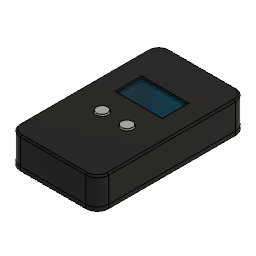
sms-telegram-enclosure (Autodesk Fusion 360 design; units mm, degrees)
part number: 2026-09-10-15-50-54-312
Autodesk Fusion 360 part; units mm, degrees
sketch "cover_outline" plane through (0, 0, 0) normal (0, 0, 1) x (1, 0, 0)
  line L0 (23, 78) -> (-23, 78)
  line L1 (-23, 78) -> (-23, 0)
  line L2 (-23, 0) -> (23, 0)
  line L3 (23, 0) -> (23, 78)
extrude "Extrude1" add sketch "cover_outline" along normal blind 2 makes body 1
fillet "Fillet1" radius 6 4 edges at (23, 0, 1) (-23, 0, 1) (-23, 78, 1) (23, 78, 1) on bodies 1
ref_plane "WorkPlane1" through (0, 0, 2) normal (0, 0, 1) x (1, 0, 0)
sketch "cover_m6" plane through (0, 0, 2) normal (0, 0, 1) x (1, 0, 0)
  circle A0 centre (-17, 72) radius 3.2
  circle A1 centre (17, 72) radius 3.2
  circle A2 centre (-17, 32) radius 3.2
  circle A3 centre (17, 32) radius 3.2
ref_plane "WorkPlane2" through (0, 0, 2) normal (0, 0, 1) x (1, 0, 0)
sketch "shell_outline" plane through (0, 0, 2) normal (0, 0, 1) x (1, 0, 0)
  line L0 (23, 78) -> (-23, 78)
  line L1 (-23, 78) -> (-23, 0)
  line L2 (-23, 0) -> (23, 0)
  line L3 (23, 0) -> (23, 78)
extrude "Extrude3" add sketch "shell_outline" along normal blind 14 separate body makes body 2
fillet "Fillet2" radius 6 4 edges at (23, 0, 9) (-23, 0, 9) (-23, 78, 9) (23, 78, 9) on bodies 2
shell "Shell1" thickness 2 removed faces 1 at (-7.6667, 50, 2) on bodies 2
ref_plane "WorkPlane3" through (0, 0, 2) normal (0, 0, 1) x (1, 0, 0)
sketch "pillars" plane through (0, 0, 2) normal (0, 0, 1) x (1, 0, 0)
  circle A0 centre (-17, 72) radius 6
  circle A1 centre (17, 72) radius 6
  circle A2 centre (-17, 32) radius 6
  circle A3 centre (17, 32) radius 6
ref_plane "WorkPlane4" through (0, 0, 2) normal (0, 0, 1) x (1, 0, 0)
sketch "insert_holes" plane through (0, 0, 2) normal (0, 0, 1) x (1, 0, 0)
  circle A0 centre (-17, 72) radius 4
  circle A1 centre (17, 72) radius 4
  circle A2 centre (-17, 32) radius 4
  circle A3 centre (17, 32) radius 4
ref_plane "WorkPlane5" through (0, 78, 0) normal (0, 1, 0) x (0, 0, 1)
sketch "usb_c" plane through (0, 78, 0) normal (0, 1, 0) x (1, 0, 0)
  line L0 (4.6, -7.9) -> (-4.6, -7.9)
  line L1 (-4.6, -7.9) -> (-4.6, -4.3)
  line L2 (-4.6, -4.3) -> (4.6, -4.3)
  line L3 (4.6, -4.3) -> (4.6, -7.9)
extrude "Extrude6" cut sketch "usb_c" along normal mid plane 3 bodies 2
ref_plane "WorkPlane6" through (0, 0, 16) normal (0, 0, 1) x (1, 0, 0)
sketch "front_ui" plane through (0, 0, 16) normal (0, 0, 1) x (1, 0, 0)
  line L0 (12.25, 58.4) -> (-12.25, 58.4)
  line L1 (-12.25, 58.4) -> (-12.25, 44.6)
  line L2 (-12.25, 44.6) -> (12.25, 44.6)
  line L3 (12.25, 44.6) -> (12.25, 58.4)
  circle A0 centre (-6.5, 32) radius 3.1
  circle A1 centre (6.5, 32) radius 3.1
extrude "Extrude7" cut sketch "front_ui" against normal blind 2.6 bodies 2
ref_plane "WorkPlane7" through (0, 0, 3.5) normal (0, 0, 1) x (1, 0, 0)
sketch "XIAO_pcb_sk" plane through (0, 0, 3.5) normal (0, 0, 1) x (1, 0, 0)
  line L0 (-10.5, 58) -> (10.5, 58)
  line L1 (10.5, 58) -> (10.5, 75.5)
  line L2 (10.5, 75.5) -> (-10.5, 75.5)
  line L3 (-10.5, 75.5) -> (-10.5, 58)
extrude "Extrude8" add sketch "XIAO_pcb_sk" along normal blind 1 separate body makes body 3
ref_plane "WorkPlane8" through (0, 0, 2.5) normal (0, 0, 1) x (1, 0, 0)
sketch "XIAO_bottom_sk" plane through (0, 0, 2.5) normal (0, 0, 1) x (1, 0, 0)
  line L0 (-9, 60) -> (9, 60)
  line L1 (9, 60) -> (9, 74)
  line L2 (9, 74) -> (-9, 74)
  line L3 (-9, 74) -> (-9, 60)
extrude "Extrude9" add sketch "XIAO_bottom_sk" along normal blind 1 separate body makes body 4
ref_plane "WorkPlane9" through (0, 0, 4.5) normal (0, 0, 1) x (1, 0, 0)
sketch "XIAO_shield_sk" plane through (0, 0, 4.5) normal (0, 0, 1) x (1, 0, 0)
  line L0 (-6, 59) -> (6, 59)
  line L1 (6, 59) -> (6, 68.5)
  line L2 (6, 68.5) -> (-6, 68.5)
  line L3 (-6, 68.5) -> (-6, 59)
extrude "Extrude10" add sketch "XIAO_shield_sk" along normal blind 2.4 separate body makes body 5
ref_plane "WorkPlane10" through (0, 0, 4.5) normal (0, 0, 1) x (1, 0, 0)
sketch "XIAO_usbc_sk" plane through (0, 0, 4.5) normal (0, 0, 1) x (1, 0, 0)
  line L0 (-4.45, 69.5) -> (4.45, 69.5)
  line L1 (4.45, 69.5) -> (4.45, 76.8)
  line L2 (4.45, 76.8) -> (-4.45, 76.8)
  line L3 (-4.45, 76.8) -> (-4.45, 69.5)
extrude "Extrude11" add sketch "XIAO_usbc_sk" along normal blind 3.2 separate body makes body 6
ref_plane "WorkPlane11" through (0, 0, 9.5) normal (0, 0, 1) x (1, 0, 0)
sketch "TFT_pcb_sk" plane through (0, 0, 9.5) normal (0, 0, 1) x (1, 0, 0)
  line L0 (-16, 38.5) -> (16, 38.5)
  line L1 (16, 38.5) -> (16, 64.5)
  line L2 (16, 64.5) -> (-16, 64.5)
  line L3 (-16, 64.5) -> (-16, 38.5)
extrude "Extrude12" add sketch "TFT_pcb_sk" along normal blind 1.2 separate body makes body 7
ref_plane "WorkPlane12" through (0, 0, 10.7) normal (0, 0, 1) x (1, 0, 0)
sketch "TFT_panel_sk" plane through (0, 0, 10.7) normal (0, 0, 1) x (1, 0, 0)
  line L0 (-15, 39.5) -> (15, 39.5)
  line L1 (15, 39.5) -> (15, 63.5)
  line L2 (15, 63.5) -> (-15, 63.5)
  line L3 (-15, 63.5) -> (-15, 39.5)
extrude "Extrude13" add sketch "TFT_panel_sk" along normal blind 3.3 separate body makes body 8
ref_plane "WorkPlane13" through (0, 0, 14) normal (0, 0, 1) x (1, 0, 0)
sketch "TFT_glass_sk" plane through (0, 0, 14) normal (0, 0, 1) x (1, 0, 0)
  line L0 (-12.05, 44.8) -> (12.05, 44.8)
  line L1 (12.05, 44.8) -> (12.05, 58.2)
  line L2 (12.05, 58.2) -> (-12.05, 58.2)
  line L3 (-12.05, 58.2) -> (-12.05, 44.8)
extrude "Extrude14" add sketch "TFT_glass_sk" along normal blind 1.2 separate body makes body 9
ref_plane "WorkPlane14" through (0, 0, 7) normal (0, 0, 1) x (1, 0, 0)
sketch "BTN_strip_sk" plane through (0, 0, 7) normal (0, 0, 1) x (1, 0, 0)
  line L0 (-10, 28) -> (10, 28)
  line L1 (10, 28) -> (10, 36)
  line L2 (10, 36) -> (-10, 36)
  line L3 (-10, 36) -> (-10, 28)
ref_plane "WorkPlane15" through (0, 0, 8.5) normal (0, 0, 1) x (1, 0, 0)
sketch "BTN_sw_next_sk" plane through (0, 0, 8.5) normal (0, 0, 1) x (1, 0, 0)
  line L0 (-10, 29) -> (-4, 29)
  line L1 (-4, 29) -> (-4, 35)
  line L2 (-4, 35) -> (-10, 35)
  line L3 (-10, 35) -> (-10, 29)
ref_plane "WorkPlane16" through (0, 0, 8.5) normal (0, 0, 1) x (1, 0, 0)
sketch "BTN_sw_ok_sk" plane through (0, 0, 8.5) normal (0, 0, 1) x (1, 0, 0)
  line L0 (4, 29) -> (10, 29)
  line L1 (10, 29) -> (10, 35)
  line L2 (10, 35) -> (4, 35)
  line L3 (4, 35) -> (4, 29)
ref_plane "WorkPlane17" through (0, 0, 13.5) normal (0, 0, 1) x (1, 0, 0)
sketch "BTN_cap_next_sk" plane through (0, 0, 13.5) normal (0, 0, 1) x (1, 0, 0)
  circle A0 centre (-7, 32) radius 2.8
ref_plane "WorkPlane18" through (0, 0, 13.5) normal (0, 0, 1) x (1, 0, 0)
sketch "BTN_cap_ok_sk" plane through (0, 0, 13.5) normal (0, 0, 1) x (1, 0, 0)
  circle A0 centre (7, 32) radius 2.8
ref_plane "WorkPlane19" through (0, 0, 2.5) normal (0, 0, 1) x (1, 0, 0)
ref_plane "WorkPlane20" through (0, 3, 0) normal (0, 1, 0) x (0, 0, 1)
ref_plane "WorkPlane21" through (0, 0, 2) normal (0, 0, 1) x (1, 0, 0)
sketch "ANT_wifi_sk" plane through (0, 0, 2) normal (0, 0, 1) x (1, 0, 0)
  line L0 (-20, 40) -> (20, 40)
  line L1 (20, 40) -> (20, 51)
  line L2 (20, 51) -> (-20, 51)
  line L3 (-20, 51) -> (-20, 40)
extrude "Extrude23" cut sketch "usb_c" along normal mid plane 8 bodies 2
ref_plane "WorkPlane22" through (0, 0, 2.5) normal (0, 0, 1) x (1, 0, 0)
sketch "SIM800L_sk" plane through (0, 0, 2.5) normal (0, 0, 1) x (1, 0, 0)
  line L0 (-18.5, 3) -> (6.5, 3)
  line L1 (6.5, 3) -> (6.5, 25.5)
  line L2 (6.5, 25.5) -> (-18.5, 25.5)
  line L3 (-18.5, 25.5) -> (-18.5, 3)
extrude "Extrude24" add sketch "SIM800L_sk" along normal blind 7 separate body makes body 10
ref_plane "WorkPlane23" through (0, 3, 0) normal (0, 1, 0) x (0, 0, 1)
sketch "CAP_bulk_sk" plane through (0, 3, 0) normal (0, 1, 0) x (1, 0, 0)
  circle A0 centre (13, -7.5) radius 5
extrude "Extrude25" add sketch "CAP_bulk_sk" along normal blind 20 separate body makes body 11
chamfer "Chamfer1" distance 0.8 angle 45 8 edges at (-21.2426, 76.2426, 16) (0, 78, 16) (21.2426, 76.2426, 16) (23, 39, 16) (21.2426, 1.7574, 16) (0, 0, 16) (-21.2426, 1.7574, 16) (-23, 39, 16) on bodies 2
ref_plane "WorkPlane24" through (0, 78, 0) normal (0, 1, 0) x (0, 0, 1)
sketch "usb_notch" plane through (0, 78, 0) normal (0, 1, 0) x (1, 0, 0)
  line L0 (-4.6, -1.5) -> (4.6, -1.5)
  line L1 (4.6, -1.5) -> (4.6, -7.9)
  line L2 (4.6, -7.9) -> (-4.6, -7.9)
  line L3 (-4.6, -7.9) -> (-4.6, -1.5)
extrude "Extrude26" cut sketch "usb_notch" along normal mid plane 8 bodies 2
ref_plane "WorkPlane25" through (0, 0, 9.3) normal (0, 0, 1) x (1, 0, 0)
sketch "tft_pocket" plane through (0, 0, 9.3) normal (0, 0, 1) x (1, 0, 0)
  line L0 (-17.5, 38.2) -> (-16.3, 38.2)
  line L1 (-16.3, 38.2) -> (-16.3, 43)
  line L2 (-16.3, 43) -> (-17.5, 43)
  line L3 (-17.5, 43) -> (-17.5, 38.2)
  line L4 (-17.5, 37) -> (-12, 37)
  line L5 (-12, 37) -> (-12, 38.2)
  line L6 (-12, 38.2) -> (-17.5, 38.2)
  line L7 (-17.5, 38.2) -> (-17.5, 37)
  line L8 (-17.5, 60) -> (-16.3, 60)
  line L9 (-16.3, 60) -> (-16.3, 64.8)
  line L10 (-16.3, 64.8) -> (-17.5, 64.8)
  line L11 (-17.5, 64.8) -> (-17.5, 60)
  line L12 (-17.5, 64.8) -> (-12, 64.8)
  line L13 (-12, 64.8) -> (-12, 66)
  line L14 (-12, 66) -> (-17.5, 66)
  line L15 (-17.5, 66) -> (-17.5, 64.8)
  line L16 (16.3, 38.2) -> (17.5, 38.2)
  line L17 (17.5, 38.2) -> (17.5, 43)
  line L18 (17.5, 43) -> (16.3, 43)
  line L19 (16.3, 43) -> (16.3, 38.2)
  line L20 (12, 37) -> (17.5, 37)
  line L21 (17.5, 37) -> (17.5, 38.2)
  line L22 (17.5, 38.2) -> (12, 38.2)
  line L23 (12, 38.2) -> (12, 37)
  line L24 (16.3, 60) -> (17.5, 60)
  line L25 (17.5, 60) -> (17.5, 64.8)
  line L26 (17.5, 64.8) -> (16.3, 64.8)
  line L27 (16.3, 64.8) -> (16.3, 60)
  line L28 (12, 64.8) -> (17.5, 64.8)
  line L29 (17.5, 64.8) -> (17.5, 66)
  line L30 (17.5, 66) -> (12, 66)
  line L31 (12, 66) -> (12, 64.8)
extrude "Extrude27" add sketch "tft_pocket" along normal blind 4.7 bodies 2
ref_plane "WorkPlane26" through (0, 0, 9.7) normal (0, 0, 1) x (1, 0, 0)
sketch "sim_ribs" plane through (0, 0, 9.7) normal (0, 0, 1) x (1, 0, 0)
  line L0 (-17, 8) -> (5, 8)
  line L1 (5, 8) -> (5, 9.2)
  line L2 (5, 9.2) -> (-17, 9.2)
  line L3 (-17, 9.2) -> (-17, 8)
  line L4 (-17, 19) -> (5, 19)
  line L5 (5, 19) -> (5, 20.2)
  line L6 (5, 20.2) -> (-17, 20.2)
  line L7 (-17, 20.2) -> (-17, 19)
extrude "Extrude28" add sketch "sim_ribs" along normal blind 4.3 bodies 2
ref_plane "WorkPlane27" through (0, 0, 12.7) normal (0, 0, 1) x (1, 0, 0)
sketch "cap_finger" plane through (0, 0, 12.7) normal (0, 0, 1) x (1, 0, 0)
  line L0 (8, 12) -> (18, 12)
  line L1 (18, 12) -> (18, 14)
  line L2 (18, 14) -> (8, 14)
  line L3 (8, 14) -> (8, 12)
extrude "Extrude29" add sketch "cap_finger" along normal blind 1.3 bodies 2
ref_plane "WorkPlane28" through (0, 0, 2) normal (0, 0, 1) x (1, 0, 0)
sketch "tft_posts" plane through (0, 0, 2) normal (0, 0, 1) x (1, 0, 0)
  line L0 (-15.75, 38.75) -> (-12.25, 38.75)
  line L1 (-12.25, 38.75) -> (-12.25, 42.25)
  line L2 (-12.25, 42.25) -> (-15.75, 42.25)
  line L3 (-15.75, 42.25) -> (-15.75, 38.75)
  line L4 (12.25, 38.75) -> (15.75, 38.75)
  line L5 (15.75, 38.75) -> (15.75, 42.25)
  line L6 (15.75, 42.25) -> (12.25, 42.25)
  line L7 (12.25, 42.25) -> (12.25, 38.75)
  line L8 (-1.75, 54.25) -> (1.75, 54.25)
  line L9 (1.75, 54.25) -> (1.75, 57.75)
  line L10 (1.75, 57.75) -> (-1.75, 57.75)
  line L11 (-1.75, 57.75) -> (-1.75, 54.25)
extrude "Extrude30" add sketch "tft_posts" along normal blind 7.4 bodies 1
ref_plane "WorkPlane29" through (0, 0, 4.6) normal (0, 0, 1) x (1, 0, 0)
sketch "xiao_hook" plane through (0, 0, 4.6) normal (0, 0, 1) x (1, 0, 0)
  line L0 (-1.75, 57.75) -> (1.75, 57.75)
  line L1 (1.75, 57.75) -> (1.75, 58.6)
  line L2 (1.75, 58.6) -> (-1.75, 58.6)
  line L3 (-1.75, 58.6) -> (-1.75, 57.75)
extrude "Extrude31" add sketch "xiao_hook" along normal blind 1 bodies 1
ref_plane "WorkPlane30" through (0, 0, 2) normal (0, 0, 1) x (1, 0, 0)
sketch "xiao_rails" plane through (0, 0, 2) normal (0, 0, 1) x (1, 0, 0)
  line L0 (-10.6, 60) -> (-9.3, 60)
  line L1 (-9.3, 60) -> (-9.3, 75)
  line L2 (-9.3, 75) -> (-10.6, 75)
  line L3 (-10.6, 75) -> (-10.6, 60)
  line L4 (9.3, 60) -> (10.6, 60)
  line L5 (10.6, 60) -> (10.6, 75)
  line L6 (10.6, 75) -> (9.3, 75)
  line L7 (9.3, 75) -> (9.3, 60)
extrude "Extrude32" add sketch "xiao_rails" along normal blind 1.5 bodies 1
ref_plane "WorkPlane31" through (0, 0, 2) normal (0, 0, 1) x (1, 0, 0)
sketch "xiao_stops" plane through (0, 0, 2) normal (0, 0, 1) x (1, 0, 0)
  line L0 (-12, 61) -> (-10.8, 61)
  line L1 (-10.8, 61) -> (-10.8, 65)
  line L2 (-10.8, 65) -> (-12, 65)
  line L3 (-12, 65) -> (-12, 61)
  line L4 (10.8, 61) -> (12, 61)
  line L5 (12, 61) -> (12, 65)
  line L6 (12, 65) -> (10.8, 65)
  line L7 (10.8, 65) -> (10.8, 61)
extrude "Extrude33" add sketch "xiao_stops" along normal blind 3.5 bodies 1
ref_plane "WorkPlane32" through (0, 0, 2) normal (0, 0, 1) x (1, 0, 0)
sketch "usb_tab" plane through (0, 0, 2) normal (0, 0, 1) x (1, 0, 0)
  line L0 (-4.5, 76) -> (4.5, 76)
  line L1 (4.5, 76) -> (4.5, 78)
  line L2 (4.5, 78) -> (-4.5, 78)
  line L3 (-4.5, 78) -> (-4.5, 76)
extrude "Extrude34" add sketch "usb_tab" along normal blind 2.2 bodies 1
ref_plane "WorkPlane33" through (0, 0, 2) normal (0, 0, 1) x (1, 0, 0)
sketch "btn_posts" plane through (0, 0, 2) normal (0, 0, 1) x (1, 0, 0)
  line L0 (-10.5, 30) -> (-6.5, 30)
  line L1 (-6.5, 30) -> (-6.5, 34)
  line L2 (-6.5, 34) -> (-10.5, 34)
  line L3 (-10.5, 34) -> (-10.5, 30)
  line L4 (6.5, 30) -> (10.5, 30)
  line L5 (10.5, 30) -> (10.5, 34)
  line L6 (10.5, 34) -> (6.5, 34)
  line L7 (6.5, 34) -> (6.5, 30)
extrude "Extrude35" add sketch "btn_posts" along normal blind 2.3 bodies 1
ref_plane "WorkPlane34" through (0, 0, 4.3) normal (0, 0, 1) x (1, 0, 0)
sketch "btn_pegs" plane through (0, 0, 4.3) normal (0, 0, 1) x (1, 0, 0)
  circle A0 centre (-8.5, 32) radius 0.9
  circle A1 centre (8.5, 32) radius 0.9
extrude "Extrude36" add sketch "btn_pegs" along normal blind 2.2 bodies 1
ref_plane "WorkPlane35" through (0, 0, 2) normal (0, 0, 1) x (1, 0, 0)
sketch "sim_stops" plane through (0, 0, 2) normal (0, 0, 1) x (1, 0, 0)
  line L0 (-20, 3) -> (-18.8, 3)
  line L1 (-18.8, 3) -> (-18.8, 8)
  line L2 (-18.8, 8) -> (-20, 8)
  line L3 (-20, 8) -> (-20, 3)
  line L4 (-20, 2) -> (-14, 2)
  line L5 (-14, 2) -> (-14, 2.7)
  line L6 (-14, 2.7) -> (-20, 2.7)
  line L7 (-20, 2.7) -> (-20, 2)
  line L8 (6.8, 3) -> (7.8, 3)
  line L9 (7.8, 3) -> (7.8, 8)
  line L10 (7.8, 8) -> (6.8, 8)
  line L11 (6.8, 8) -> (6.8, 3)
  line L12 (2, 2) -> (7.8, 2)
  line L13 (7.8, 2) -> (7.8, 2.7)
  line L14 (7.8, 2.7) -> (2, 2.7)
  line L15 (2, 2.7) -> (2, 2)
  line L16 (-20, 21) -> (-18.8, 21)
  line L17 (-18.8, 21) -> (-18.8, 25.5)
  line L18 (-18.8, 25.5) -> (-20, 25.5)
  line L19 (-20, 25.5) -> (-20, 21)
  line L20 (6.8, 21) -> (7.8, 21)
  line L21 (7.8, 21) -> (7.8, 25.5)
  line L22 (7.8, 25.5) -> (6.8, 25.5)
  line L23 (6.8, 25.5) -> (6.8, 21)
  line L24 (-12, 25.8) -> (-1, 25.8)
  line L25 (-1, 25.8) -> (-1, 26.6)
  line L26 (-1, 26.6) -> (-12, 26.6)
  line L27 (-12, 26.6) -> (-12, 25.8)
extrude "Extrude37" add sketch "sim_stops" along normal blind 3 bodies 1
ref_plane "WorkPlane36" through (0, 0, 2) normal (0, 0, 1) x (1, 0, 0)
sketch "cap_saddles" plane through (0, 0, 2) normal (0, 0, 1) x (1, 0, 0)
  line L0 (7.5, 4.5) -> (18.5, 4.5)
  line L1 (18.5, 4.5) -> (18.5, 6.5)
  line L2 (18.5, 6.5) -> (7.5, 6.5)
  line L3 (7.5, 6.5) -> (7.5, 4.5)
  line L4 (7.5, 19.5) -> (18.5, 19.5)
  line L5 (18.5, 19.5) -> (18.5, 21.5)
  line L6 (18.5, 21.5) -> (7.5, 21.5)
  line L7 (7.5, 21.5) -> (7.5, 19.5)
extrude "Extrude38" add sketch "cap_saddles" along normal blind 5.5 bodies 1
ref_plane "WorkPlane37" through (0, 3, 0) normal (0, 1, 0) x (0, 0, 1)
sketch "cap_saddle_cut" plane through (0, 3, 0) normal (0, 1, 0) x (1, 0, 0)
  circle A0 centre (13, -7.5) radius 5.2
extrude "Extrude39" cut sketch "cap_saddle_cut" along normal blind 20 bodies 1
ref_plane "WorkPlane38" through (0, 0, 4) normal (0, 0, 1) x (1, 0, 0)
sketch "btn_strip_holes" plane through (0, 0, 4) normal (0, 0, 1) x (1, 0, 0)
  circle A0 centre (-8.5, 32) radius 1
  circle A1 centre (8.5, 32) radius 1
ref_plane "WorkPlane39" through (0, 0, 2) normal (0, 0, 1) x (1, 0, 0)
sketch "ANT_wifi_sk2" plane through (0, 0, 2) normal (0, 0, 1) x (1, 0, 0)
  line L0 (-20, 42.5) -> (20, 42.5)
  line L1 (20, 42.5) -> (20, 53.5)
  line L2 (20, 53.5) -> (-20, 53.5)
  line L3 (-20, 53.5) -> (-20, 42.5)
extrude "Extrude41" add sketch "ANT_wifi_sk2" along normal blind 1 separate body makes body 12
combine "Combine1" operation cut target body 1 tool bodies 2 keep tools
ref_plane "WorkPlane40" through (0, 0, 4.3) normal (0, 0, 1) x (1, 0, 0)
sketch "BTN_strip_sk (1)" plane through (0, 0, 4.3) normal (0, 0, 1) x (1, 0, 0)
  line L0 (-10, 28) -> (10, 28)
  line L1 (10, 28) -> (10, 36)
  line L2 (10, 36) -> (-10, 36)
  line L3 (-10, 36) -> (-10, 28)
extrude "Extrude42" add sketch "BTN_strip_sk (1)" along normal blind 1.6 separate body makes body 13
ref_plane "WorkPlane41" through (0, 0, 4) normal (0, 0, 1) x (1, 0, 0)
sketch "BTN_strip_holes2" plane through (0, 0, 4) normal (0, 0, 1) x (1, 0, 0)
  circle A0 centre (-8.5, 32) radius 1
  circle A1 centre (8.5, 32) radius 1
extrude "Extrude43" cut sketch "BTN_strip_holes2" along normal blind 2.5 bodies 13
ref_plane "WorkPlane42" through (0, 0, 5.9) normal (0, 0, 1) x (1, 0, 0)
sketch "BTN_sw_next_sk (1)" plane through (0, 0, 5.9) normal (0, 0, 1) x (1, 0, 0)
  line L0 (-9.5, 29) -> (-3.5, 29)
  line L1 (-3.5, 29) -> (-3.5, 35)
  line L2 (-3.5, 35) -> (-9.5, 35)
  line L3 (-9.5, 35) -> (-9.5, 29)
extrude "Extrude44" add sketch "BTN_sw_next_sk (1)" along normal blind 3.5 separate body makes body 14
ref_plane "WorkPlane43" through (0, 0, 9.4) normal (0, 0, 1) x (1, 0, 0)
sketch "BTN_sw_next_plunger" plane through (0, 0, 9.4) normal (0, 0, 1) x (1, 0, 0)
  circle A0 centre (-6.5, 32) radius 1.75
extrude "Extrude45" add sketch "BTN_sw_next_plunger" along normal blind 3.5 bodies 14
ref_plane "WorkPlane44" through (0, 0, 5.9) normal (0, 0, 1) x (1, 0, 0)
sketch "BTN_sw_ok_sk (1)" plane through (0, 0, 5.9) normal (0, 0, 1) x (1, 0, 0)
  line L0 (3.5, 29) -> (9.5, 29)
  line L1 (9.5, 29) -> (9.5, 35)
  line L2 (9.5, 35) -> (3.5, 35)
  line L3 (3.5, 35) -> (3.5, 29)
extrude "Extrude46" add sketch "BTN_sw_ok_sk (1)" along normal blind 3.5 separate body makes body 15
ref_plane "WorkPlane45" through (0, 0, 9.4) normal (0, 0, 1) x (1, 0, 0)
sketch "BTN_sw_ok_plunger" plane through (0, 0, 9.4) normal (0, 0, 1) x (1, 0, 0)
  circle A0 centre (6.5, 32) radius 1.75
extrude "Extrude47" add sketch "BTN_sw_ok_plunger" along normal blind 3.5 bodies 15
ref_plane "WorkPlane46" through (0, 0, 13) normal (0, 0, 1) x (1, 0, 0)
sketch "BTN_cap_next_sk (1)" plane through (0, 0, 13) normal (0, 0, 1) x (1, 0, 0)
  circle A0 centre (-6.5, 32) radius 4
extrude "Extrude48" add sketch "BTN_cap_next_sk (1)" along normal blind 1 separate body makes body 16
ref_plane "WorkPlane47" through (0, 0, 14) normal (0, 0, 1) x (1, 0, 0)
sketch "BTN_cap_next_stem" plane through (0, 0, 14) normal (0, 0, 1) x (1, 0, 0)
  circle A0 centre (-6.5, 32) radius 2.8
extrude "Extrude49" add sketch "BTN_cap_next_stem" along normal blind 2.8 bodies 16
ref_plane "WorkPlane48" through (0, 0, 13) normal (0, 0, 1) x (1, 0, 0)
sketch "BTN_cap_next_socket" plane through (0, 0, 13) normal (0, 0, 1) x (1, 0, 0)
  circle A0 centre (-6.5, 32) radius 1.85
extrude "Extrude50" cut sketch "BTN_cap_next_socket" along normal blind 1 bodies 16
ref_plane "WorkPlane49" through (0, 0, 13) normal (0, 0, 1) x (1, 0, 0)
sketch "BTN_cap_ok_sk (1)" plane through (0, 0, 13) normal (0, 0, 1) x (1, 0, 0)
  circle A0 centre (6.5, 32) radius 4
extrude "Extrude51" add sketch "BTN_cap_ok_sk (1)" along normal blind 1 separate body makes body 17
ref_plane "WorkPlane50" through (0, 0, 14) normal (0, 0, 1) x (1, 0, 0)
sketch "BTN_cap_ok_stem" plane through (0, 0, 14) normal (0, 0, 1) x (1, 0, 0)
  circle A0 centre (6.5, 32) radius 2.8
extrude "Extrude52" add sketch "BTN_cap_ok_stem" along normal blind 2.8 bodies 17
ref_plane "WorkPlane51" through (0, 0, 13) normal (0, 0, 1) x (1, 0, 0)
sketch "BTN_cap_ok_socket" plane through (0, 0, 13) normal (0, 0, 1) x (1, 0, 0)
  circle A0 centre (6.5, 32) radius 1.85
extrude "Extrude53" cut sketch "BTN_cap_ok_socket" along normal blind 1 bodies 17
ref_plane "WorkPlane52" through (0, 0, 5.7) normal (0, 0, 1) x (1, 0, 0)
sketch "peg_trim" plane through (0, 0, 5.7) normal (0, 0, 1) x (1, 0, 0)
  line L0 (-12, 27) -> (12, 27)
  line L1 (12, 27) -> (12, 37)
  line L2 (12, 37) -> (-12, 37)
  line L3 (-12, 37) -> (-12, 27)
extrude "Extrude54" cut sketch "peg_trim" along normal blind 2 bodies 1
ref_plane "WorkPlane80" through (0, 0, 3.4) normal (0, 0, 1) x (1, 0, 0)
sketch "pillars_m3" plane through (0, 0, 3.4) normal (0, 0, 1) x (1, 0, 0)
  circle A0 centre (-17.8, 32) radius 4
  circle A1 centre (-17.8, 72) radius 4
  circle A2 centre (17.8, 32) radius 4
  circle A3 centre (17.8, 72) radius 4
extrude "Extrude82" add sketch "pillars_m3" along normal blind 10.6 bodies 2
ref_plane "WorkPlane81" through (0, 0, 3.4) normal (0, 0, 1) x (1, 0, 0)
sketch "insert_holes_m3" plane through (0, 0, 3.4) normal (0, 0, 1) x (1, 0, 0)
  circle A0 centre (-17.8, 32) radius 2.2
  circle A1 centre (-17.8, 72) radius 2.2
  circle A2 centre (17.8, 32) radius 2.2
  circle A3 centre (17.8, 72) radius 2.2
extrude "Extrude83" cut sketch "insert_holes_m3" along normal blind 6 bodies 2
ref_plane "WorkPlane82" through (0, 0, 2) normal (0, 0, 1) x (1, 0, 0)
sketch "boss_m3_0" plane through (0, 0, 2) normal (0, 0, 1) x (1, 0, 0)
  circle A0 centre (-17.8, 32) radius 4
  line L0 (-20.7, 27) -> (-20.7, 37)
extrude "Extrude84" add sketch "boss_m3_0" along normal blind 1.4 contours A0 L0 picked at (-17.6978, 33.1513) bodies 1
ref_plane "WorkPlane83" through (0, 0, 2) normal (0, 0, 1) x (1, 0, 0)
sketch "boss_m3_1" plane through (0, 0, 2) normal (0, 0, 1) x (1, 0, 0)
  circle A0 centre (-17.8, 72) radius 4
  line L0 (-20.7, 67) -> (-20.7, 77)
extrude "Extrude85" add sketch "boss_m3_1" along normal blind 1.4 contours A0 L0 picked at (-18.1062, 72) bodies 1
ref_plane "WorkPlane84" through (0, 0, 2) normal (0, 0, 1) x (1, 0, 0)
sketch "boss_m3_2" plane through (0, 0, 2) normal (0, 0, 1) x (1, 0, 0)
  circle A0 centre (17.8, 32) radius 4
  line L0 (20.7, 27) -> (20.7, 37)
extrude "Extrude86" add sketch "boss_m3_2" along normal blind 1.4 contours A0 L0 picked at (18.7466, 32.9138) bodies 1
ref_plane "WorkPlane85" through (0, 0, 2) normal (0, 0, 1) x (1, 0, 0)
sketch "boss_m3_3" plane through (0, 0, 2) normal (0, 0, 1) x (1, 0, 0)
  circle A0 centre (17.8, 72) radius 4
  line L0 (20.7, 67) -> (20.7, 77)
extrude "Extrude87" add sketch "boss_m3_3" along normal blind 1.4 contours A0 L0 picked at (18.4, 72) bodies 1
ref_plane "WorkPlane86" through (0, 0, 0) normal (0, 0, 1) x (1, 0, 0)
sketch "cover_thru_m3" plane through (0, 0, 0) normal (0, 0, 1) x (1, 0, 0)
  circle A0 centre (-17.8, 32) radius 1.7
  circle A1 centre (-17.8, 72) radius 1.7
  circle A2 centre (17.8, 32) radius 1.7
  circle A3 centre (17.8, 72) radius 1.7
extrude "Extrude88" cut sketch "cover_thru_m3" along normal blind 3.4 bodies 1
ref_plane "WorkPlane87" through (0, 0, 0) normal (0, 0, 1) x (1, 0, 0)
sketch "counterbore_m3" plane through (0, 0, 0) normal (0, 0, 1) x (1, 0, 0)
  circle A0 centre (-17.8, 32) radius 3.1
  circle A1 centre (-17.8, 72) radius 3.1
  circle A2 centre (17.8, 32) radius 3.1
  circle A3 centre (17.8, 72) radius 3.1
extrude "Extrude89" cut sketch "counterbore_m3" along normal blind 1.9 bodies 1
ref_plane "WorkPlane88" through (0, 0, 3.4) normal (0, 0, 1) x (1, 0, 0)
sketch "INSERT_0_sk" plane through (0, 0, 3.4) normal (0, 0, 1) x (1, 0, 0)
  circle A0 centre (-17.8, 32) radius 2.2
extrude "Extrude90" add sketch "INSERT_0_sk" along normal blind 5 separate body makes body 18
ref_plane "WorkPlane89" through (0, 0, 3.4) normal (0, 0, 1) x (1, 0, 0)
sketch "INSERT_0_bore" plane through (0, 0, 3.4) normal (0, 0, 1) x (1, 0, 0)
  circle A0 centre (-17.8, 32) radius 1.5
extrude "Extrude91" cut sketch "INSERT_0_bore" along normal blind 5 bodies 18
ref_plane "WorkPlane90" through (0, 0, 0.25) normal (0, 0, 1) x (1, 0, 0)
sketch "SCREW_0_head" plane through (0, 0, 0.25) normal (0, 0, 1) x (1, 0, 0)
  circle A0 centre (-17.8, 32) radius 2.85
extrude "Extrude92" add sketch "SCREW_0_head" along normal blind 1.65 separate body makes body 19
ref_plane "WorkPlane91" through (0, 0, 1.9) normal (0, 0, 1) x (1, 0, 0)
sketch "SCREW_0_shank" plane through (0, 0, 1.9) normal (0, 0, 1) x (1, 0, 0)
  circle A0 centre (-17.8, 32) radius 1.45
extrude "Extrude93" add sketch "SCREW_0_shank" along normal blind 6 bodies 19
ref_plane "WorkPlane92" through (0, 0, 3.4) normal (0, 0, 1) x (1, 0, 0)
sketch "INSERT_1_sk" plane through (0, 0, 3.4) normal (0, 0, 1) x (1, 0, 0)
  circle A0 centre (-17.8, 72) radius 2.2
extrude "Extrude94" add sketch "INSERT_1_sk" along normal blind 5 separate body makes body 20
ref_plane "WorkPlane93" through (0, 0, 3.4) normal (0, 0, 1) x (1, 0, 0)
sketch "INSERT_1_bore" plane through (0, 0, 3.4) normal (0, 0, 1) x (1, 0, 0)
  circle A0 centre (-17.8, 72) radius 1.5
extrude "Extrude95" cut sketch "INSERT_1_bore" along normal blind 5 bodies 20
ref_plane "WorkPlane94" through (0, 0, 0.25) normal (0, 0, 1) x (1, 0, 0)
sketch "SCREW_1_head" plane through (0, 0, 0.25) normal (0, 0, 1) x (1, 0, 0)
  circle A0 centre (-17.8, 72) radius 2.85
extrude "Extrude96" add sketch "SCREW_1_head" along normal blind 1.65 separate body makes body 21
ref_plane "WorkPlane95" through (0, 0, 1.9) normal (0, 0, 1) x (1, 0, 0)
sketch "SCREW_1_shank" plane through (0, 0, 1.9) normal (0, 0, 1) x (1, 0, 0)
  circle A0 centre (-17.8, 72) radius 1.45
extrude "Extrude97" add sketch "SCREW_1_shank" along normal blind 6 bodies 21
ref_plane "WorkPlane96" through (0, 0, 3.4) normal (0, 0, 1) x (1, 0, 0)
sketch "INSERT_2_sk" plane through (0, 0, 3.4) normal (0, 0, 1) x (1, 0, 0)
  circle A0 centre (17.8, 32) radius 2.2
extrude "Extrude98" add sketch "INSERT_2_sk" along normal blind 5 separate body makes body 22
ref_plane "WorkPlane97" through (0, 0, 3.4) normal (0, 0, 1) x (1, 0, 0)
sketch "INSERT_2_bore" plane through (0, 0, 3.4) normal (0, 0, 1) x (1, 0, 0)
  circle A0 centre (17.8, 32) radius 1.5
extrude "Extrude99" cut sketch "INSERT_2_bore" along normal blind 5 bodies 22
ref_plane "WorkPlane98" through (0, 0, 0.25) normal (0, 0, 1) x (1, 0, 0)
sketch "SCREW_2_head" plane through (0, 0, 0.25) normal (0, 0, 1) x (1, 0, 0)
  circle A0 centre (17.8, 32) radius 2.85
extrude "Extrude100" add sketch "SCREW_2_head" along normal blind 1.65 separate body makes body 23
ref_plane "WorkPlane99" through (0, 0, 1.9) normal (0, 0, 1) x (1, 0, 0)
sketch "SCREW_2_shank" plane through (0, 0, 1.9) normal (0, 0, 1) x (1, 0, 0)
  circle A0 centre (17.8, 32) radius 1.45
extrude "Extrude101" add sketch "SCREW_2_shank" along normal blind 6 bodies 23
ref_plane "WorkPlane100" through (0, 0, 3.4) normal (0, 0, 1) x (1, 0, 0)
sketch "INSERT_3_sk" plane through (0, 0, 3.4) normal (0, 0, 1) x (1, 0, 0)
  circle A0 centre (17.8, 72) radius 2.2
extrude "Extrude102" add sketch "INSERT_3_sk" along normal blind 5 separate body makes body 24
ref_plane "WorkPlane101" through (0, 0, 3.4) normal (0, 0, 1) x (1, 0, 0)
sketch "INSERT_3_bore" plane through (0, 0, 3.4) normal (0, 0, 1) x (1, 0, 0)
  circle A0 centre (17.8, 72) radius 1.5
extrude "Extrude103" cut sketch "INSERT_3_bore" along normal blind 5 bodies 24
ref_plane "WorkPlane102" through (0, 0, 0.25) normal (0, 0, 1) x (1, 0, 0)
sketch "SCREW_3_head" plane through (0, 0, 0.25) normal (0, 0, 1) x (1, 0, 0)
  circle A0 centre (17.8, 72) radius 2.85
extrude "Extrude104" add sketch "SCREW_3_head" along normal blind 1.65 separate body makes body 25
ref_plane "WorkPlane103" through (0, 0, 1.9) normal (0, 0, 1) x (1, 0, 0)
sketch "SCREW_3_shank" plane through (0, 0, 1.9) normal (0, 0, 1) x (1, 0, 0)
  circle A0 centre (17.8, 72) radius 1.45
extrude "Extrude105" add sketch "SCREW_3_shank" along normal blind 6 bodies 25
combine "Combine2" operation cut target body 1 tool bodies 2 keep tools
equation "ow = 46 mm" comment "outer width X"
equation "oh = 78 mm" comment "outer length Y"
equation "od = 16 mm" comment "outer depth Z"
equation "wall = 2.0 mm" comment "wall"
equation "cover_t = 2.0 mm" comment "bottom cover thickness"
equation "insert_hole = 4.4 mm" comment "M6 brass heat-set insert hole (Notion inventory)"
equation "pillar_od = 8.0 mm" comment "M6 pillar OD (2 mm around insert)"
equation "cover_hole = 3.4 mm" comment "M6 clearance"
equation "corner_r = 6.0 mm" comment "outer corner R = pillar R"
named bodies: "BottomCover", "UpperShell", "XIAO_pcb", "XIAO_bottom", "XIAO_shield", "XIAO_usbc", "TFT_pcb", "TFT_panel", "TFT_glass", "SIM800L", "CAP_bulk", "ANT_wifi", "BTN_strip", "BTN_sw_next", "BTN_sw_ok", "BTN_cap_next", "BTN_cap_ok", "INSERT_0", "SCREW_0", "INSERT_1", "SCREW_1", "INSERT_2", "SCREW_2", "INSERT_3", "SCREW_3"
